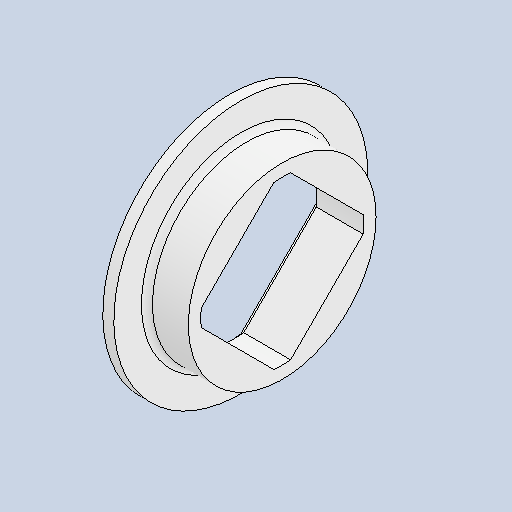
# Autodesk Inventor part: joint3_washer2
Saved by Autodesk Inventor 2025.3 (Build 293356030, 356C)
## iProperties
Created: 2025-11-20
Part Number: joint3_washer2
Material: PLA filament
Document SubType Name: Modeling
Designer: MSI
Mass: 6.25446 g
Surface Area: 41.101 cm^2
Volume: 5.21205 cm^3
Density: 1.2 g/cm^3
Appearance: 일반
Author: MSI
Autodesk Inventor part; units mm, degrees
ref_plane "YZ Plane" through (0, 0, 0) normal (1, 0, 0) x (0, 1, 0)
ref_plane "XZ Plane" through (0, 0, 0) normal (0, 1, 0) x (-1, 0, 0)
ref_plane "XY Plane" through (0, 0, 0) normal (0, 0, 1) x (1, 0, 0)
sketch "스케치1" plane through (0, 0, 0) normal (1, 0, 0) x (0, 1, 0)
  circle A0 centre (0, 0) radius 23
  dimension "d0" = 46
  constraints: 1 centre point, 1 coincident
  measures "d0" diameter of A0
extrude "돌출1" add sketch "스케치1" along normal blind 2
sketch "스케치2" plane through (2, 0, 0) normal (1, 0, 0) x (0, 0, -1)
  circle A0 centre (0, 0) radius 23 projected
  constraints: 1 coincident
hole "구멍1" at (2, 0, 0) direction (-1, 0, 0) diameter 29.5 end through all
sketch "스케치3" plane through (2, 0, 0) normal (1, 0, 0) x (0, 0, -1)
  circle A0 centre (0, 0) radius 14.75 projected
  circle A1 centre (0, 0) radius 17
  dimension "d14" = 34
  constraints: 1 centre point
  measures "d14" diameter of A1
extrude "돌출2" add sketch "스케치3" along normal blind 7.5
fillet "모깎기1" radius 1 1 edges at (2, 0, 17)
sketch "스케치4" plane through (9.5, 0, 0) normal (1, 0, 0) x (0, 0, -1)
  circle A0 centre (0, 0) radius 14.75 projected
  line L0 (0, -16.1927) -> (16.1927, 0)
  line L1 (16.1927, 0) -> (0, 16.1927)
  line L2 (0, 16.1927) -> (-16.1927, 0)
  line L3 (-16.1927, 0) -> (0, -16.1927)
  line L4 (0, -16.1927) -> (0, 16.1927) construction
  line L5 (16.1927, 0) -> (-16.1927, 0) construction
  point P0 (-1.5214, -14.6713)
  point P1 (-14.6713, -1.5214)
  point P2 (-14.6713, 1.5214)
  point P3 (-1.5214, 14.6713)
  point P4 (1.5214, 14.6713)
  point P5 (14.6713, 1.5214)
  point P6 (1.5214, -14.6713)
  point P7 (14.6713, -1.5214)
  dimension "d15" = 22.9
  dimension "d16" = 22.9
  constraints: 12 end point, 2 midpoint, 2 parallel, 1 perpendicular, 1 vertical
  measures "d15" distance of L0.start L0.end
  measures "d16" distance of L0.end L1.end
extrude "돌출3" add sketch "스케치4" against normal up to surface (9.5 mm away) contours A0 L1 L0 | L1 A0 | A0 L0 | A0 L2 L1 | L0 L3 A0 | L2 A0 | A0 L3 | A0 L3 L2
chamfer "모따기1" distance 1 angle 45 8 edges at (0, -8.0964, -8.0964) (0, 0, -14.75) (0, 14.75, 0) (0, 8.0964, 8.0964) (0, 0, 14.75) (0, -14.75, 0) (0, -8.0964, 8.0964) (0, 8.0964, -8.0964)
equation "\"d16\" = d15"
equation "\"joint4_belt_centor\" = 157.367"
equation "\"joint4_axis2_L\" = 58.803"
equation "\"joint4_axis2_b1\" = 35"
equation "\"joint4_axis2_d\" = 19"
equation "\"joint4_miter_m\" = 2"
equation "\"joint4_miter_a\" = 20deg"
equation "\"joint4_miter_z\" = 79"
equation "\"joint4_miter_b\" = 6.90139"
equation "\"joint4_axis3_L\" = 23.5"
equation "\"joint3_belt_centor\" = 157.367"
equation "\"joint3_axis2_L\" = 63.75"
equation "\"joint3_axis2_b1\" = 38"
equation "\"joint3_axis2_d\" = 29"
equation "\"joint3_planetary_m\" = 2"
equation "\"joint3_planetary_a\" = 20deg"
equation "\"joint3_planetary_np\" = 4"
equation "\"joint3_sun_b\" = 19"
equation "\"joint3_planet_b\" = 19"
equation "\"joint3_ring_b\" = 18"
equation "\"joint3_axis3_d\" = 29"
equation "\"joint3_miter_m\" = 4"
equation "\"joint3_miter_a\" = 20deg"
equation "\"joint3_miter_z1\" = 26"
equation "\"joint3_miter_z2\" = 39"
equation "\"joint3_miter_b\" = 25.07657"
equation "\"joint3_axis4_L\" = 43.706"
